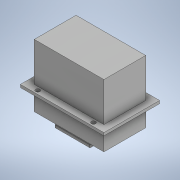
# Autodesk Inventor part: Servo
Saved by Autodesk Inventor 2022 (Build 260153000, 153)
## iProperties
Created: 2022-01-13
Part Number: Servo
Material: Generic
Document SubType Name: Modeling
Designer: nguye
Density: 1 g/cm^3
Appearance: Default
Author: nguye
Autodesk Inventor part; units mm, degrees
ref_plane "YZ Plane" through (0, 0, 0) normal (1, 0, 0) x (0, 1, 0)
ref_plane "XZ Plane" through (0, 0, 0) normal (0, 1, 0) x (-1, 0, 0)
ref_plane "XY Plane" through (0, 0, 0) normal (0, 0, 1) x (1, 0, 0)
sketch "Sketch1" plane through (0, 0, 0) normal (0, 1, 0) x (-1, 0, 0)
  line L0 (0, 0) -> (50, 0)
  line L1 (50, 0) -> (50, -30)
  line L2 (50, -30) -> (0, -30)
  line L3 (0, -30) -> (0, 0)
  dimension "d0" = 50
  dimension "d1" = 30
  constraints: 8 end point, 2 parallel, 1 horizontal, 1 perpendicular
  measures "d0" distance of L1.end L2.end
  measures "d1" distance of L0.end L1.end
extrude "Extrusion1" add sketch "Sketch1" along normal blind 50
sketch "Sketch2" plane through (0, 50, 0) normal (0, 1, 0) x (1, 0, 0)
  line L0 (5, -5) -> (-55, -5)
  line L1 (-55, -5) -> (-55, 35)
  line L2 (-55, 35) -> (5, 35)
  line L3 (5, 35) -> (5, -5)
  point P0 (0, 0)
  dimension "d4" = 60
  dimension "d5" = 40
  constraints: 8 end point, 2 parallel, 1 horizontal, 1 perpendicular
  measures "d4" distance of L1.end L2.end
  measures "d5" distance of L0.end L1.end
extrude "Extrusion2" add sketch "Sketch2" against normal blind 30
sketch "Sketch3" plane through (0, 50, 0) normal (0, 1, 0) x (1, 0, 0)
  line L0 (0, 0) -> (0, 30) projected
  line L1 (0, 30) -> (-50, 30) projected
  line L2 (0, 0) -> (-50, 0)
  line L3 (-50, 0) -> (-50, 30)
  line L4 (-50, 30) -> (0, 30)
  line L5 (0, 30) -> (0, 0)
  line L6 (5, -5) -> (-55, -5) projected
  line L7 (-55, -5) -> (-55, 35) projected
  line L8 (5, -5) -> (-55, -5)
  line L9 (-55, -5) -> (-55, 35)
  line L10 (-55, 35) -> (5, 35)
  line L11 (5, 35) -> (5, -5)
  dimension "d8" = 50
  dimension "d9" = 30
  constraints: 16 end point, 4 parallel, 2 horizontal, 2 perpendicular
  measures "d8" distance of L1.end L4.end
  measures "d9" distance of L2.end L1.end
extrude "Extrusion3" cut sketch "Sketch3" against normal blind 28
sketch "Sketch4" plane through (0, 0, 0) normal (0, -1, 0) x (1, 0, 0)
  line L0 (-50, 0) -> (0, 0) projected
  line L1 (0, -30) -> (-50, -30) projected
  line L2 (0, 0) -> (-50, 0)
  line L3 (-50, 0) -> (-50, -30)
  line L4 (-50, -30) -> (0, -30)
  line L5 (0, -30) -> (0, 0)
  constraints: 8 end point, 2 parallel, 1 horizontal, 1 perpendicular
extrude "Extrusion4" cut sketch "Sketch4" against normal blind 5
sketch "Sketch5" plane through (0, 5, 0) normal (0, -1, 0) x (1, 0, 0)
  circle A0 centre (-25, -15) radius 2.5
  point P0 (0, 0)
  dimension "d14" = 5
  constraints: 1 centre point
  measures "d14" diameter of A0
extrude "Extrusion5" add sketch "Sketch5" along normal blind 3
sketch "Sketch6" plane through (-25, 2, -15) normal (0, -1, 0) x (1, 0, 0)
  line L0 (-12.5, 12.5) -> (12.5, 12.5)
  line L1 (12.5, 12.5) -> (12.5, -12.5)
  line L2 (12.5, -12.5) -> (-12.5, -12.5)
  line L3 (-12.5, -12.5) -> (-12.5, 12.5)
  circle A0 centre (-10, 10) radius 1.5
  circle A1 centre (-10, -10) radius 1.5
  circle A2 centre (10, -10) radius 1.5
  circle A3 centre (10, 10) radius 1.5
  point P0 (25, 15)
  dimension "d19" = 25
  dimension "d20" = 25
  dimension "d21" = 3
  dimension "d22" = 3
  dimension "d23" = 3
  dimension "d24" = 3
  constraints: 8 end point, 4 centre point, 2 parallel, 1 horizontal, 1 perpendicular
  measures "d19" distance of L1.end L2.end
  measures "d20" distance of L0.end L1.end
  measures "d21" diameter of A0
  measures "d22" diameter of A1
  measures "d23" diameter of A2
  measures "d24" diameter of A3
extrude "Extrusion6" add sketch "Sketch6" along normal blind 2
sketch "Sketch7" plane through (-25, 0, -15) normal (0, -1, 0) x (1, 0, 0)
  circle A0 centre (0, 0) radius 2.5
  point P0 (25, 15)
  dimension "d27" = 5
  constraints: 1 centre point
  measures "d27" diameter of A0
extrude "Extrusion7" add sketch "Sketch7" along normal blind 3
sketch "Sketch8" plane through (0, 20, 0) normal (0, -1, 0) x (1, 0, 0)
  line L0 (-50, -30) -> (-50, 0) projected
  circle A0 centre (-5, -32.5) radius 1.5
  circle A1 centre (-5, 2.5) radius 1.5
  circle A2 centre (-45, 2.5) radius 1.5
  circle A3 centre (-45, -32.5) radius 1.5
  point P0 (0, 0)
  point P1 (0, -30)
  dimension "d38" = 3
  dimension "d39" = 3
  dimension "d40" = 3
  dimension "d41" = 3
  constraints: 4 centre point
  measures "d38" diameter of A0
  measures "d39" diameter of A1
  measures "d40" diameter of A2
  measures "d41" diameter of A3
extrude "Extrusion8" cut sketch "Sketch8" against normal blind 3
body "Solid1"
